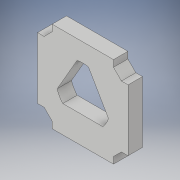
# Autodesk Inventor part: 20_IM_Cube_Insert_Lens_holder_RMS_63x
Saved by Autodesk Inventor 2019 (Build 230136000, 136)
## iProperties
Created: 2019-10-23
Part Number: 20_IM_Cube_Insert_Lens_holder_RMS_63x
Material: Generic
Document SubType Name: Modeling
Designer: marsikovabarbora
Density: 1 g/cm^3
Appearance: Default
Lens_diameter: 25,000 mm
Author: marsikovabarbora
Autodesk Inventor part; units mm, degrees
ref_plane "YZ Plane" through (0, 0, 0) normal (1, 0, 0) x (0, 1, 0)
ref_plane "XZ Plane" through (0, 0, 0) normal (0, 1, 0) x (-1, 0, 0)
ref_plane "XY Plane" through (0, 0, 0) normal (0, 0, 1) x (1, 0, 0)
sketch "Sketch1" plane through (0, 0, 0) normal (0, 0, 1) x (1, 0, 0)
  line L0 (-35.2109, 0) -> (35.2109, 0) construction
  line L1 (0, -35.2109) -> (0, 35.2109) construction
  line L2 (0, 0) -> (13.4339, 13.4339) construction
  line L3 (0, 0) -> (18.9985, 0) construction
  line L4 (0, 25.1006) -> (17, 25.1006)
  line L5 (17, 25.1006) -> (17, 21.4406)
  line L6 (17, 21.4406) -> (19.2203, 19.2203)
  line L7 (25.1006, 0) -> (25.1006, 17)
  line L8 (25.1006, 17) -> (21.4406, 17)
  line L9 (21.4406, 17) -> (19.2203, 19.2203)
  line L10 (0, 0) -> (-13.4339, 13.4339) construction
  line L11 (0, 0) -> (-18.9985, 0) construction
  line L12 (0, 25.1006) -> (-17, 25.1006)
  line L13 (-17, 25.1006) -> (-17, 21.4406)
  line L14 (-17, 21.4406) -> (-19.2203, 19.2203)
  line L15 (-25.1006, 0) -> (-25.1006, 17)
  line L16 (-25.1006, 17) -> (-21.4406, 17)
  line L17 (-21.4406, 17) -> (-19.2203, 19.2203)
  line L18 (0, 0) -> (13.4339, -13.4339) construction
  line L19 (0, -25.1006) -> (17, -25.1006)
  line L20 (17, -25.1006) -> (17, -21.4406)
  line L21 (17, -21.4406) -> (19.2203, -19.2203)
  line L22 (25.1006, 0) -> (25.1006, -17)
  line L23 (25.1006, -17) -> (21.4406, -17)
  line L24 (21.4406, -17) -> (19.2203, -19.2203)
  line L25 (0, 0) -> (-13.4339, -13.4339) construction
  line L26 (0, -25.1006) -> (-17, -25.1006)
  line L27 (-17, -25.1006) -> (-17, -21.4406)
  line L28 (-17, -21.4406) -> (-19.2203, -19.2203)
  line L29 (-25.1006, 0) -> (-25.1006, -17)
  line L30 (-25.1006, -17) -> (-21.4406, -17)
  line L31 (-21.4406, -17) -> (-19.2203, -19.2203)
  line L32 (-17.05, 25.1506) -> (0, 25.1506)
  line L33 (0, 25.1506) -> (17.05, 25.1506)
  line L34 (17.05, 25.1506) -> (17.05, 21.4613)
  line L35 (17.05, 21.4613) -> (19.2557, 19.2557)
  line L36 (19.2557, 19.2557) -> (21.4613, 17.05)
  line L37 (21.4613, 17.05) -> (25.1506, 17.05)
  line L38 (25.1506, 17.05) -> (25.1506, 0)
  line L39 (25.1506, 0) -> (25.1506, -17.05)
  line L40 (25.1506, -17.05) -> (21.4613, -17.05)
  line L41 (21.4613, -17.05) -> (19.2557, -19.2557)
  line L42 (19.2557, -19.2557) -> (17.05, -21.4613)
  line L43 (17.05, -21.4613) -> (17.05, -25.1506)
  line L44 (17.05, -25.1506) -> (0, -25.1506)
  line L45 (0, -25.1506) -> (-17.05, -25.1506)
  line L46 (-17.05, -25.1506) -> (-17.05, -21.4613)
  line L47 (-17.05, -21.4613) -> (-19.2557, -19.2557)
  line L48 (-19.2557, -19.2557) -> (-21.4613, -17.05)
  line L49 (-21.4613, -17.05) -> (-25.1506, -17.05)
  line L50 (-25.1506, -17.05) -> (-25.1506, 0)
  line L51 (-25.1506, 0) -> (-25.1506, 17.05)
  line L52 (-25.1506, 17.05) -> (-21.4613, 17.05)
  line L53 (-21.4613, 17.05) -> (-19.2557, 19.2557)
  line L54 (-19.2557, 19.2557) -> (-17.05, 21.4613)
  line L55 (-17.05, 21.4613) -> (-17.05, 25.1506)
  dimension "d0" = 45
  dimension "d1" = 3.14
  dimension "d2" = 3.66
  dimension "d3" = 17
  dimension "d23" = 0.05
  constraints: 108 end point, 24 symmetric about line, 5 point on line, 3 perpendicular, 2 horizontal, 1 equal length, 23 other
  measures "d0" angle of L3 L2
  measures "d1" distance of L5.end L6.end
  measures "d2" distance of L4.end L5.end
  measures "d3" distance of L4.start L4.end
  measures "d23" distance between parallel lines of L12 L32
extrude "Extrusion1" add sketch "Sketch1" along normal blind 8 contours L4 L5 L6 L9 L8 L7 L22 L23 L24 L21 L20 L19 L26 L27 L28 L31 L30 L29 L15 L16 L17 L14 L13 L12 | L32 L33 L34 L35 L36 L37 L38 L39 L40 L41 L42 L43 L44 L45 L46 L47 L48 L49 L50 L51 L52 L53 L54 L55
hole "Hole1" at (0, 0, 0) direction (0, 0, 1) diameter 30 end through all
sketch "Sketch2" plane through (0, 0, 0) normal (0, 0, -1) x (-1, 0, 0)
  circle A0 centre (0, 0) radius 15 projected
  line L0 (3.1688, 14.6615) -> (14.2816, -4.5865)
  line L1 (11.1128, -10.075) -> (-11.1128, -10.075)
  line L2 (-14.2816, -4.5865) -> (-3.1688, 14.6615)
  circle A1 centre (0, 0) radius 10.075 construction
  circle A2 centre (0, 0) radius 15 construction
  circle A3 centre (0, 0) radius 15 construction
  arc A4 (14.2816, -4.5865) -> (3.1688, 14.6615) centre (0, 0) ccw
  arc A5 (-11.1128, -10.075) -> (11.1128, -10.075) centre (0, 0) ccw
  arc A6 (-3.1688, 14.6615) -> (-14.2816, -4.5865) centre (0, 0) ccw
  dimension "d22" = 20.15
  constraints: 7 point on circle, 6 end point, 4 centre point, 2 coincident, 1 point on line, 1 tangent, 16 other
  measures "d22" diameter of A1
extrude "Extrusion2" add sketch "Sketch2" against normal up to surface (8 mm away) contours A0 L0 | L2 A0 | A0 L1
equation "\"Lens_diameter\" = 25"
body "Solid1"
